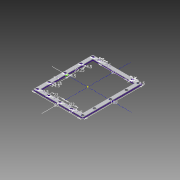
# Autodesk Inventor part: Side
Saved by Autodesk Inventor 2014 SP1 (Build 180222100, 222)
## iProperties
Created: 2015-03-28
Part Number: Side
Material: ABS Plastic
Document SubType Name: Modeling
Designer: Erin
Density: 1.06 g/cm^3
Appearance: Smooth - White
Mass: 2.88336 g
Surface Area: 49.7096 cm^2
Volume: 2.72015 cm^3
Author: Erin
Autodesk Inventor part; units mm, degrees
ref_plane "YZ Plane" through (0, 0, 0) normal (1, 0, 0) x (0, 1, 0)
ref_plane "XZ Plane" through (0, 0, 0) normal (0, 1, 0) x (-1, 0, 0)
ref_plane "XY Plane" through (0, 0, 0) normal (0, 0, 1) x (1, 0, 0)
sketch "Sketch1" plane through (0, 0, 0) normal (0, 0, 1) x (1, 0, 0)
  line L0 (-41.5, 50) -> (41.5, 50)
  line L1 (41.5, 50) -> (41.5, -50)
  line L2 (41.5, -50) -> (-41.5, -50)
  line L3 (-41.5, -50) -> (-41.5, 50)
  line L4 (35.5, 44) -> (-35.5, 44)
  line L5 (-35.5, 44) -> (-35.5, -44)
  line L6 (-35.5, -44) -> (35.5, -44)
  line L7 (35.5, -44) -> (35.5, 44)
  line L8 (-41.5, -47) -> (41.5, -47) construction
  circle A0 centre (-19.75, -47) radius 2.25
  line L9 (0, 71.7466) -> (0, -78.0681) construction
  circle A1 centre (0, -47) radius 2.25
  circle A2 centre (19.75, -47) radius 2.25
  line L10 (-60.2597, 0) -> (74.2823, 0) construction
  line L11 (-38.5, 50) -> (-38.5, -50) construction
  circle A3 centre (-38.5, 0) radius 2.25
  circle A4 centre (-38.5, 27) radius 2.25
  circle A5 centre (-38.5, -27) radius 2.25
  line L12 (-41.5, 47) -> (41.5, 47) construction
  line L13 (-35.5, -3) -> (-35.5, 3)
  circle A6 centre (-38.5, 47) radius 2.25
  circle A7 centre (-38.5, -47) radius 2.25
  line L14 (-25, 50) -> (25, 50)
  line L15 (25, 50) -> (25, 47)
  line L16 (25, 47) -> (-25, 47)
  line L17 (-25, 47) -> (-25, 50)
  circle A8 centre (-28, 47) radius 2.25
  circle A9 centre (28, 47) radius 2.25
  point P0 (0, 0)
  point P1 (0, 50)
  point P2 (41.5, 0)
  point P3 (0, 47)
  point P4 (0, 47)
  dimension "d0" = 83
  dimension "d1" = 100
  dimension "d2" = 4.5
  dimension "d3" = 4.5
  dimension "d4" = 4.5
  dimension "d5" = 3
  dimension "d6" = 3
  dimension "d9" = 3
  dimension "d10" = 4.5
  dimension "d11" = 4.5
  dimension "d12" = 4.5
  dimension "d17" = 3
  dimension "d41" = 4.5
  dimension "d42" = 4.5
  dimension "d45" = 29.25
  dimension "d46" = 29.25
  dimension "d47" = 22
  dimension "d48" = 22
  dimension "d66" = 50
  dimension "d67" = 3
  dimension "d81" = 4.5
  dimension "d82" = 4.5
  dimension "d83" = 3
  dimension "d84" = 3
  constraints: 36 end point, 19 point on line, 10 centre point, 8 perpendicular, 6 midpoint, 6 parallel, 3 horizontal, 2 vertical alignment, 1 horizontal alignment, 1 vertical, 3 other
  measures "d0" distance of L1.end L2.end
  measures "d1" distance of L0.end L1.end
  measures "d2" diameter of A0
  measures "d3" diameter of A1
  measures "d4" diameter of A2
  measures "d5" distance between parallel lines of L8 L2
  measures "d6" distance between parallel lines of L6 L8
  measures "d9" distance between parallel lines of L11 L3
  measures "d10" diameter of A3
  measures "d11" diameter of A4
  measures "d12" diameter of A5
  measures "d17" distance between parallel lines of L12 L0
  measures "d41" diameter of A6
  measures "d42" diameter of A7
  measures "d66" distance of L15.end L16.end
  measures "d67" distance of L14.end L15.end
  measures "d81" diameter of A8
  measures "d82" diameter of A9
  measures "d83" distance from line of A8.centre L17
  measures "d84" distance from line of A9.centre L15
extrude "Extrusion1" add sketch "Sketch1" along normal blind 1.5 contours L0 L17 L16 L15 L1 L2 L3 | L0 L15 L16 L17 | A3 | A4 | A5 | A6 | A7 | A8 | A9
extrude "Extrusion2" cut sketch "Sketch1" along normal blind 10 contours A3 | A4 | A5 | A6 | A7
mirror "Mirror1" about plane through (0, 0, 0) normal (1, 0, 0) of "Extrusion2"
extrude "Extrusion7" cut sketch "Sketch1" along normal blind 10 contours A8 | A9
body "Solid1"
